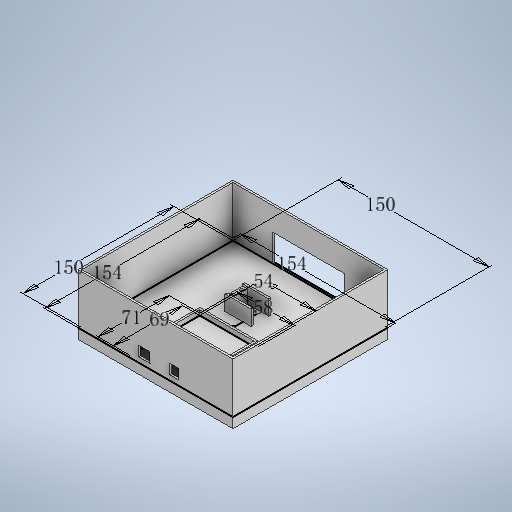
# Autodesk Inventor part: 底座
Saved by Autodesk Inventor 2025 (Build 290162000, 162)
## iProperties
Created: 2024-03-30
Part Number: 底座
Material: 常规
Document SubType Name: Modeling
Designer: Huijun Wang
Density: 1 g/cm^3
Appearance: 默认
Author: Huijun Wang
Autodesk Inventor part; units mm, degrees
ref_plane "YZ Plane" through (0, 0, 0) normal (1, 0, 0) x (0, 1, 0)
ref_plane "XZ Plane" through (0, 0, 0) normal (0, 1, 0) x (-1, 0, 0)
ref_plane "XY Plane" through (0, 0, 0) normal (0, 0, 1) x (1, 0, 0)
sketch "草图1" plane through (0, 0, 0) normal (0, 1, 0) x (-1, 0, 0)
  line L0 (77, 77) -> (-77, 77)
  line L1 (-77, 77) -> (-77, -77)
  line L2 (-77, -77) -> (77, -77)
  line L3 (77, -77) -> (77, 77)
  line L4 (0, 0) -> (0, -24)
  line L5 (0, 0) -> (17, 0)
  line L6 (75, 75) -> (-75, 75)
  line L7 (-75, 75) -> (-75, -75)
  line L8 (-75, -75) -> (75, -75)
  line L9 (75, -75) -> (75, 75)
  line L10 (-27, 6) -> (27, 6)
  line L11 (29, 4) -> (-29, 4)
  line L12 (29, 4) -> (29, 75)
  line L13 (-29, 4) -> (-29, 75)
  line L14 (27, 6) -> (27, 75)
  line L15 (-27, 6) -> (-27, 75)
  dimension "d1" = 154
  dimension "d2" = 154
  dimension "d3" = 150
  dimension "d4" = 150
  dimension "d5" = 54
  dimension "d6" = 58
  dimension "d7" = 71
  dimension "d8" = 69
  constraints: 32 end point, 6 perpendicular, 5 horizontal, 4 parallel, 4 point on line, 1 vertical, 6 other
  measures "d1" distance of L1.end L2.end
  measures "d2" distance of L2.end L0.start
  measures "d3" distance of L7.end L8.end
  measures "d4" distance of L8.end L6.start
  measures "d5" distance of L10.start L10.end
  measures "d6" distance of L11.start L11.end
  measures "d7" distance of L11.start L12.end
  measures "d8" distance of L10.end L14.end
sketch "草图4" plane through (0, 0, 0) normal (0, 1, 0) x (-1, 0, 0)
  line L0 (77, 77) -> (-77, 77)
  line L1 (-77, 77) -> (-77, -77)
  line L2 (-77, -77) -> (77, -77)
  line L3 (77, -77) -> (77, 77)
  line L4 (0, 0) -> (0, -178.4057)
  line L5 (0, 0) -> (-63.1988, 0)
  line L6 (75, 75) -> (-75, 75)
  line L7 (-75, 75) -> (-75, -75)
  line L8 (-75, -75) -> (75, -75)
  line L9 (75, -75) -> (75, 75)
  line L10 (-27, 6) -> (27, 6)
  line L11 (29, 4) -> (-29, 4)
  line L12 (29, 4) -> (29, 75)
  line L13 (-29, 4) -> (-29, 75)
  line L14 (27, 6) -> (27, 75)
  line L15 (-27, 6) -> (-27, 75)
  dimension "d11" = 154
  dimension "d12" = 154
  dimension "d13" = 150
  dimension "d14" = 150
  dimension "d15" = 54
  dimension "d16" = 58
  dimension "d17" = 71
  dimension "d18" = 69
  constraints: 32 end point, 6 perpendicular, 5 horizontal, 4 parallel, 4 point on line, 1 coincident, 1 vertical, 6 other
  measures "d11" distance of L1.end L2.end
  measures "d12" distance of L2.end L0.start
  measures "d13" distance of L7.end L8.end
  measures "d14" distance of L8.end L6.start
  measures "d15" distance of L10.start L10.end
  measures "d16" distance of L11.start L11.end
  measures "d17" distance of L11.start L12.end
  measures "d18" distance of L10.end L14.end
sketch "草图5" plane through (0, 0, 0) normal (0, 1, 0) x (-1, 0, 0)
  line L0 (77, 77) -> (-77, 77)
  line L1 (-77, 77) -> (-77, -77)
  line L2 (-77, -77) -> (77, -77)
  line L3 (77, -77) -> (77, 77)
  line L4 (0, 0) -> (0, -24)
  line L5 (0, 0) -> (17, 0)
  line L6 (75, 75) -> (-75, 75)
  line L7 (-75, 75) -> (-75, -75)
  line L8 (-75, -75) -> (75, -75)
  line L9 (75, -75) -> (75, 75)
  line L10 (-27, 6) -> (27, 6)
  line L11 (29, 4) -> (-29, 4)
  line L12 (29, 4) -> (29, 75)
  line L13 (-29, 4) -> (-29, 75)
  line L14 (27, 6) -> (27, 75)
  line L15 (-27, 6) -> (-27, 75)
  dimension "d19" = 154
  dimension "d20" = 154
  dimension "d21" = 150
  dimension "d22" = 150
  dimension "d23" = 54
  dimension "d24" = 58
  dimension "d25" = 71
  dimension "d26" = 69
  constraints: 32 end point, 6 perpendicular, 5 horizontal, 4 parallel, 4 point on line, 1 coincident, 1 vertical, 6 other
  measures "d19" distance of L1.end L2.end
  measures "d20" distance of L2.end L0.start
  measures "d21" distance of L7.end L8.end
  measures "d22" distance of L8.end L6.start
  measures "d23" distance of L10.start L10.end
  measures "d24" distance of L11.start L11.end
  measures "d25" distance of L11.start L12.end
  measures "d26" distance of L10.end L14.end
sketch "草图6" plane through (0, 0, 0) normal (0, 1, 0) x (-1, 0, 0)
  line L0 (0, 0) -> (0, -24)
  line L1 (0, 0) -> (17, 0)
  line L2 (-75, 75) -> (-75, -75)
  line L3 (-77, 77) -> (-77, -77)
  line L4 (29, 4) -> (-29, 4)
  line L5 (-27, 6) -> (27, 6)
  line L6 (75, 75) -> (-75, 75)
  line L7 (77, 77) -> (-77, 77)
  line L8 (29, 4) -> (29, 75)
  line L9 (27, 6) -> (27, 75)
  line L10 (-29, 4) -> (-29, 75)
  line L11 (-27, 6) -> (-27, 75)
  line L12 (-77, -77) -> (77, -77)
  line L13 (-75, -75) -> (75, -75)
  line L14 (77, -77) -> (77, 77)
  line L15 (75, -75) -> (75, 75)
  dimension "d27" = 154
  dimension "d28" = 154
  dimension "d29" = 150
  dimension "d30" = 150
  dimension "d31" = 54
  dimension "d32" = 58
  dimension "d33" = 71
  dimension "d34" = 69
  constraints: 32 end point, 6 perpendicular, 5 horizontal, 4 parallel, 4 point on line, 2 coincident, 1 vertical, 6 other
  measures "d27" distance of L3.end L12.end
  measures "d28" distance of L12.end L7.start
  measures "d29" distance of L2.end L13.end
  measures "d30" distance of L13.end L6.start
  measures "d31" distance of L5.start L5.end
  measures "d32" distance of L4.start L4.end
  measures "d33" distance of L4.start L8.end
  measures "d34" distance of L5.end L9.end
extrude "拉伸2" add sketch "草图4" along normal blind 5 contours L3 L2 L1 L0 | L6 L15 L10 L14 L12 L11 L13
extrude "拉伸3" add sketch "草图1" against normal blind 10 contours L3 L2 L1 L0 | L9 L8 L7 L6 L13 L11 L12 | L12 L11 L13 L6 L15 L10 L14 | L14 L10 L15 L6
extrude "拉伸4" add sketch "草图5" along normal blind 50
sketch "草图7" plane through (-77, -10, 77) normal (0, 0, 1) x (1, 0, 0)
  line L0 (77, 10) -> (104, 10)
  line L1 (2, 10) -> (152, 10) projected
  line L2 (104, 10) -> (104, 25)
  line L3 (104, 25) -> (50, 25)
  line L4 (50, 25) -> (50, 10)
  line L5 (50, 10) -> (104, 10)
  line L6 (77, 10) -> (77, 15)
  line L7 (77, 15) -> (50, 15)
  line L8 (60, 15) -> (60, 25)
  line L9 (60, 25) -> (50, 25)
  line L10 (60, 25) -> (50, 25)
  line L11 (60, 25) -> (71.5, 25)
  line L12 (71.5, 25) -> (71.5, 15)
  line L13 (50, 25) -> (91, 25)
  line L14 (50, 25) -> (100, 25)
  line L15 (91, 25) -> (91, 15)
  line L16 (91, 15) -> (100, 15)
  line L17 (100, 15) -> (100, 25)
  dimension "d42" = 15
  dimension "d43" = 54
  dimension "d44" = 5
  dimension "d45" = 10
  dimension "d46" = 10
  dimension "d47" = 11.5
  dimension "d48" = 41
  dimension "d49" = 50
  dimension "d50" = 10
  constraints: 34 end point, 9 point on line, 8 perpendicular, 2 collinear, 2 vertical
  measures "d42" distance of L0.end L2.end
  measures "d43" distance of L2.end L3.end
  measures "d44" distance of L0.start L6.end
  measures "d45" distance of L8.start L8.end
  measures "d46" distance of L3.end L8.end
  measures "d47" distance of L8.end L11.end
  measures "d48" distance of L3.end L13.end
  measures "d49" distance of L3.end L14.end
  measures "d50" distance of L13.end L15.end
extrude "拉伸5" cut sketch "草图7" against normal blind 3 contours L7 L8 L3 L12 | L17 L16 L15 L3
sketch "草图8" plane through (77, -10, -77) normal (0, 0, -1) x (-1, 0, 0)
  line L0 (77, 10) -> (112.5, 10)
  line L1 (50, 10) -> (104, 10) projected
  line L2 (112.5, 10) -> (112.5, 37)
  line L3 (112.5, 37) -> (41.5, 37)
  line L4 (41.5, 37) -> (41.5, 10)
  line L5 (41.5, 10) -> (77, 10)
  dimension "d53" = 35.5
  dimension "d54" = 27
  dimension "d55" = 71
  constraints: 10 end point, 4 perpendicular, 1 collinear, 1 point on line
  measures "d53" distance of L0.start L0.end
  measures "d54" distance of L0.end L2.end
  measures "d55" distance of L2.end L3.end
extrude "拉伸6" cut sketch "草图8" against normal blind 3
sketch "草图9" plane through (0, 0, 0) normal (0, 1, 0) x (1, 0, 0)
  line L0 (0, 0) -> (0, 10)
  line L1 (0, 10) -> (-18, 10)
  line L2 (0, 10) -> (8, 10)
  line L3 (8, 10) -> (8, 12)
  line L4 (8, 12) -> (-18, 12)
  line L5 (-18, 12) -> (-18, 10)
  line L6 (0, 12) -> (0, 27.6)
  line L7 (0, 27.6) -> (-18, 27.6)
  line L8 (-18, 27.6) -> (-18, 29.6)
  line L9 (-18, 29.6) -> (8, 29.6)
  line L10 (8, 29.6) -> (8, 27.6)
  line L11 (8, 27.6) -> (0, 27.6)
  line L12 (-18, 27.6) -> (-18, 12)
  line L13 (-18, 12) -> (-13, 12)
  line L14 (-13, 12) -> (-13, 27.6)
  line L15 (-18, 27.6) -> (-13, 27.6)
  dimension "d58" = 10
  dimension "d59" = 18
  dimension "d60" = 8
  dimension "d61" = 15.6
  dimension "d62" = 2
  dimension "d75" = 5
  constraints: 32 end point, 10 perpendicular, 3 point on line, 2 horizontal, 2 vertical, 1 collinear
  measures "d58" distance of L0.start L0.end
  measures "d59" distance of L0.end L1.end
  measures "d60" distance of L0.end L2.end
  measures "d61" distance of L6.start L6.end
  measures "d62" distance of L7.end L8.end
  measures "d75" distance of L4.end L13.end
extrude "拉伸8" add sketch "草图9" along normal blind 15 contours L1 L5 L4 L3 L2 | L12 L7 L14 L4 | L8 L9 L10 L11 L7
sketch "草图14" plane through (0, 15, 0) normal (0, 1, 0) x (1, 0, 0)
  line L0 (-13, 12) -> (-13, 27.6) projected
  line L1 (-13, 27.6) -> (-13, 12)
  line L2 (-13, 12) -> (-18, 12)
  line L3 (-18, 12) -> (-18, 27.6)
  line L4 (-18, 27.6) -> (-13, 27.6)
  point P0 (0, 0)
  constraints: 8 end point, 3 perpendicular, 1 vertical
extrude "拉伸9" cut sketch "草图14" against normal blind 2
sketch "草图15" plane through (0, 13, 0) normal (0, 1, 0) x (1, 0, 0)
  line L0 (-18, 27.6) -> (8, 27.6) projected
  line L1 (-18, 27.6) -> (-15.5, 27.6)
  line L2 (-15.5, 27.6) -> (-15.5, 23.8)
  line L3 (-15.5, 23.8) -> (-15.5, 15.8)
  circle A0 centre (-15.5, 23.8) radius 1.5
  circle A1 centre (-15.5, 15.8) radius 1.5
  point P0 (0, 0)
  dimension "d80" = 2.5
  dimension "d81" = 3.8
  dimension "d82" = 8
  dimension "d83" = 3
  dimension "d84" = 3
  constraints: 6 end point, 2 centre point, 2 coincident, 2 point on line, 1 perpendicular
  measures "d80" distance of L0.start L1.end
  measures "d81" distance of L1.end L2.end
  measures "d82" distance of L2.end L3.end
  measures "d83" diameter of A0
  measures "d84" diameter of A1
extrude "拉伸10" cut sketch "草图15" against normal blind 13
